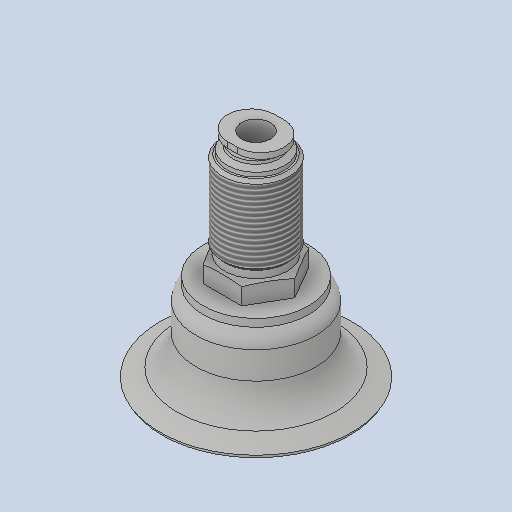
# Autodesk Inventor part: MVFKN40-1-1
Saved by Autodesk Inventor 2024.1 (Build 281209000, 209)
## iProperties
Category: PARTsolutions
Company: MISUMI
Created: 2023-12-16
Part Number: MVFKN40-1-1
Material: Generic
Catalog Web Link: www.cadenas.de
Description: MVPKN, MVPKE, MVPKF, MVFKN, MVFKF,MVSKS_1-Suction Cups - StandardType, Deep Type, Sponge Type - Fixed Type Up: One  - Touch Type (K Shape)_1
Vendor: MISUMI
Document SubType Name: Modeling
Designer: psAdmin
Manufacturer: MISUMI
Mass: 14.6095 g
Surface Area: 52.8765 cm^2
Volume: 14.6095 cm^3
Density: 1 g/cm^3
Appearance: PSOLRGB-175-175-175
PSOL_IDENT_0: {$CADENAS_DATA/23d-libs/misumi/metric/35_tubes_nozzles/mvpkn/mvpkn.prj},200 {VTYP=3D},{NB=MVFKN40-1-
PSOL_IDENT_1: 1},{LINA=MVFKN40-1},{NN=MVPKN, MVPKE, MVPKF, MVFKN, MVFKF,MVSKS_1},{DATE=04.06.2021 06:55:05},{GEOMD
PSOL_IDENT_2: ATE=14.07.2014 08:56:00},{VERSION=},{LINEID=120},{WBVAR=MATP},{WBNUMERIC=}  {NB=MVFKN40-1-1},{LINA=M
PSOL_IDENT_3: VFKN40-1},{KT=DUMMY},{PN=MVFKN40-1},{MATM=Brass},{TYPE=MVFKN},{ST=Electroless Nickel Plating},{AC=Su
PSOL_IDENT_4: ction Cup},{SHAPE=Deep},{MATP=N},{MATPALG='N', 'Nitrile Rubber','F','Fluoro Rubber'},{NL1=40 - 17.5}
PSOL_IDENT_5: ,{NO=40},{NO1=40},{D=6},{DD=40},{L1=17.5},{B=45.2},{L2=23.1},{L3=18.0},{H1=17},{T=4},{M=M14x1.0},{M1=
PSOL_IDENT_6: 14},{M2=1.00},{L4=11.7},{MASS=47.0},{TIFF=2},{MVPNT=1},{MVPFT=1},{K1=0},{K2=0},{K3=0.0},{MVPKN=1},{P
PSOL_IDENT_7: LANE=17.500},{R1=4.9},{H2=7.0},{H3=9.5},{H4=12.0},{L5=0.0},{L6=1.5},{H5=22.0},{H6=14},{VD1=40},{VD2=
PSOL_IDENT_8: 25.0},{VD3=0.0},{VH1=17.5},{VH2=4.5},{VX1=0.00},{VX2=0.0},{VY1=0.77},{VY2=0.0},{VY3=0.00},{VR1=7.00}
NB: MVFKN40-1-1
NN: MVPKN, MVPKE, MVPKF, MVFKN, MVFKF,MVSKS_1
NT: Suction Cups - StandardType, Deep Type, Sponge Type - Fixed Type Up: One  - Touch Type (K Shape)_1
NBSYN: $PN.-1
LINA: MVFKN40-1
CATALOG: Misumi
PN: MVFKN40-1
MATM: Brass
ST: Electroless Nickel Plating
AC: Suction Cup
SHAPE: Deep
MATP: Nitrile Rubber
NL1: 40 - 17.5
NO: 40
D: 6
DD: 40
L1: 17.5
B: 45.2
L2: 23.1
L3: 18
H1: 17
T: 4
M: M14x1.0
M2: 1
MASS: 47
K1: 0
K2: 0
K3: 0
PLANE: 17.5
R1: 4.9
H2: 7
H3: 9.5
H4: 12
L5: 0
L6: 1.5
H5: 22
H6: 14
VD1: 40
VD2: 25
VD3: 0
VH1: 17.5
VH2: 4.5
VX1: 0
VX2: 0
VY1: 0.77
VY2: 0
VY3: 0
VR1: 7
SUPPLIER: MISUMI
ARTICLENO: MVFKN40-1-1
BOMINFO: MVFKN40-1
CREATOR: CADENAS GmbH
Title: MVFKN40-1
Author: Cadenas PARTsolutions
Comments: Suction Cups - StandardType, Deep Type, Sponge Type - Fixed Type Up: One  - Touch Type (K Shape)_1
Autodesk Inventor part; units mm, degrees
sketch "Sketch_1" plane through (0, 45.2, 0) normal (0, 1, 0) x (1, 0, 0)
  arc A0 (-1, 4.9) -> (-1, -4.9) centre (-1, 0) ccw
  line L0 (-1, -4.9) -> (1, -4.9)
  arc A1 (1, -4.9) -> (1, 4.9) centre (1, 0) ccw
  line L1 (1, 4.9) -> (-1, 4.9)
  constraints: 4 end point, 4 point on circle, 2 centre point
extrude "Extrusion1" add sketch "Sketch_1" against normal blind 1.2
sketch "Sketch_2" plane through (0, 0, 0) normal (0, 0, 1) x (1, 0, 0)
  line L0 (0, 41.1) -> (0, 44)
  line L1 (0, 44) -> (3.5, 44)
  line L2 (3.5, 44) -> (3.5, 43.1)
  line L3 (3.5, 43.1) -> (4.75, 43.1)
  line L4 (4.75, 43.1) -> (4.884, 42.6)
  line L5 (4.884, 42.6) -> (6, 41.9557)
  line L6 (6, 41.9557) -> (6, 41.1)
  line L7 (6, 41.1) -> (0, 41.1)
  line L8 (0, 41.1) -> (0, 44)
  constraints: 18 end point
revolve "Revolution1" add sketch "Sketch_2" angle 360 about axis through (0, 41.1, 0) along (0, -1, 0)
sketch "Sketch_5" plane through (0, 0, 0) normal (0, 0, 1) x (1, 0, 0)
  line L0 (0, 24.6) -> (0, 41.1)
  line L1 (0, 41.1) -> (6.3865, 41.1)
  line L2 (6.3865, 41.1) -> (7, 40.4865)
  line L3 (7, 40.4865) -> (7, 25.2135)
  line L4 (7, 25.2135) -> (6.3865, 24.6)
  line L5 (6.3865, 24.6) -> (0, 24.6)
  line L6 (0, 24.6) -> (0, 41.1)
  constraints: 14 end point
revolve "Revolution2" add sketch "Sketch_5" angle 360 about axis through (0, 24.6, 0) along (0, -1, 0)
thread "Thread1" size "M14x1" class "6g" standard "ISO Metric profile" full length
sketch "Sketch_6" plane through (0, 0, 0) normal (0, 0, 1) x (1, 0, 0)
  line L0 (0, 23.1) -> (0, 24.6)
  line L1 (0, 24.6) -> (6.5, 24.6)
  line L2 (6.5, 24.6) -> (6.5, 23.1)
  line L3 (6.5, 23.1) -> (0, 23.1)
  line L4 (0, 23.1) -> (0, 24.6)
  constraints: 10 end point
revolve "Revolution3" add sketch "Sketch_6" angle 360 about axis through (0, 23.1, 0) along (0, -1, 0)
sketch "Sketch_8" plane through (0, 0, 0) normal (0, 0, 1) x (1, 0, 0)
  line L0 (0, 17.5) -> (0, 23.1)
  line L1 (0, 23.1) -> (6, 23.1)
  line L2 (6, 23.1) -> (8.4, 22.4569)
  line L3 (8.4, 22.4569) -> (8.4, 18.1431)
  line L4 (8.4, 18.1431) -> (6, 17.5)
  line L5 (6, 17.5) -> (0, 17.5)
  line L6 (0, 17.5) -> (0, 23.1)
  constraints: 14 end point
revolve "Revolution4" add sketch "Sketch_8" angle 360 about axis through (0, 17.5, 0) along (0, -1, 0)
sketch "Sketch_9" plane through (0, 23.1, 0) normal (0, 1, 0) x (1, 0, 0)
  line L0 (-12, -12) -> (12, -12)
  line L1 (12, -12) -> (12, 12)
  line L2 (12, 12) -> (-12, 12)
  line L3 (-12, 12) -> (-12, -12)
  line L4 (-8.0829, 0) -> (-4.0415, -7)
  line L5 (-4.0415, -7) -> (4.0415, -7)
  line L6 (4.0415, -7) -> (8.0829, 0)
  line L7 (8.0829, 0) -> (4.0415, 7)
  line L8 (4.0415, 7) -> (-4.0415, 7)
  line L9 (-4.0415, 7) -> (-8.0829, 0)
  constraints: 20 end point
extrude "Extrusion2" cut sketch "Sketch_9" against normal blind 5.6
sketch "Sketch_10" plane through (0, 0, 0) normal (0, 0, 1) x (1, 0, 0)
  line L0 (0, 17.5) -> (0, 19.1)
  line L1 (0, 19.1) -> (11, 19.1)
  line L2 (11, 19.1) -> (11, 17.5)
  line L3 (11, 17.5) -> (0, 17.5)
  line L4 (0, 17.5) -> (0, 19.1)
  constraints: 10 end point
revolve "Revolution5" add sketch "Sketch_10" angle 360 about axis through (0, 17.5, 0) along (0, -1, 0)
sketch "Sketch_12" plane through (0, 0, 0) normal (0, 0, 1) x (1, 0, 0)
  line L0 (0, 33.5) -> (0, 45.2)
  line L1 (0, 45.2) -> (3, 45.2)
  line L2 (3, 45.2) -> (3, 33.5)
  line L3 (3, 33.5) -> (0, 33.5)
  line L4 (0, 33.5) -> (0, 45.2)
  constraints: 10 end point
revolve "Revolution6" cut sketch "Sketch_12" angle 360 about axis through (0, 33.5, 0) along (0, -1, 0)
sketch "Sketch_22" plane through (0, 0, 0) normal (0, 0, 1) x (1, 0, 0)
  line L0 (0, 17.5) -> (0, 0)
  line L1 (0, 0) -> (-19.5554, 0)
  line L2 (-19.5554, 0) -> (-20, 0.77)
  line L3 (-20, 0.77) -> (-16.3829, 2.5689)
  arc A0 (-16.3829, 2.5689) -> (-12.5, 8.8366) centre (-19.5, 8.8366) ccw
  line L4 (-12.5, 8.8366) -> (-12.5, 14.5)
  arc A1 (-9.5, 17.5) -> (-12.5, 14.5) centre (-9.5, 14.5) ccw
  line L5 (-9.5, 17.5) -> (0, 17.5)
  line L6 (0, 17.5) -> (0, 0)
  constraints: 14 end point, 4 point on circle, 2 centre point
revolve "Revolution7" add sketch "Sketch_22" angle 360 about axis through (0, 17.5, 0) along (0, 1, 0)
ref_plane "BODY_TO_PARTS_XY" through (0, 17.5, 0) normal (0, 1, 0) x (1, 0, 0)
ref_plane "BODY_TO_PARTS_YZ" through (0, 17.5, 0) normal (1, 0, 0) x (0, 0, -1)
ref_plane "BODY_TO_PARTS_ZX" through (0, 17.5, 0) normal (0, 0, -1) x (0, 1, 0)
ref_plane "body_to_nut1_XY" through (0, 30.3, 0) normal (0, 1, 0) x (1, 0, 0)
ref_plane "body_to_nut1_YZ" through (0, 30.3, 0) normal (1, 0, 0) x (0, 0, -1)
ref_plane "body_to_nut1_ZX" through (0, 30.3, 0) normal (0, 0, -1) x (0, 1, 0)
ref_plane "body_to_nut2_XY" through (0, 24.7, 0) normal (0, 1, 0) x (1, 0, 0)
ref_plane "body_to_nut2_YZ" through (0, 24.7, 0) normal (1, 0, 0) x (0, 0, -1)
ref_plane "body_to_nut2_ZX" through (0, 24.7, 0) normal (0, 0, -1) x (0, 1, 0)
ref_plane "body_to_nut3_XY" through (0, 34.6, 0) normal (0, 1, 0) x (1, 0, 0)
ref_plane "body_to_nut3_YZ" through (0, 34.6, 0) normal (1, 0, 0) x (0, 0, -1)
ref_plane "body_to_nut3_ZX" through (0, 34.6, 0) normal (0, 0, -1) x (0, 1, 0)
ref_plane "body_to_nut4_XY" through (0, 27.6, 0) normal (0, 1, 0) x (1, 0, 0)
ref_plane "body_to_nut4_YZ" through (0, 27.6, 0) normal (1, 0, 0) x (0, 0, -1)
ref_plane "body_to_nut4_ZX" through (0, 27.6, 0) normal (0, 0, -1) x (0, 1, 0)
ref_plane "作業平面17" through (0, 0, 10) normal (0, 0, 1) x (1, 0, 0)
sketch "スケッチ11" plane through (0, 0, 10) normal (0, 0, 1) x (1, 0, 0)
  arc A0 (-16.3829, 2.5689) -> (-12.5, 8.8366) centre (-19.5, 8.8366) ccw projected
  line L0 (0, 0) -> (-19.5554, 0) projected
  line L1 (-19.5554, 0) -> (-20, 0.77) projected
  line L2 (-5.9, 44) -> (-1, 44) projected
  line L3 (-1, 45.2) -> (-5.9, 45.2) projected
  line L4 (-1, 45.2) -> (-1, 44) projected
  line L5 (-4.884, 42.6) -> (4.884, 42.6) projected
  line L6 (-4.884, 42.6) -> (4.884, 42.6) projected
  line L7 (-4.75, 43.1) -> (4.75, 43.1) projected
  line L8 (-3.5, 43.1) -> (3.5, 43.1) projected
  line L9 (-4.75, 43.1) -> (4.75, 43.1) projected
  line L10 (-1, 44) -> (1, 44) projected
  line L11 (1, 44) -> (-1, 44) projected
  line L12 (3.5, 44) -> (-3.5, 44) projected
  line L13 (-3.5, 43.1) -> (3.5, 43.1) projected
  line L14 (3.5, 44) -> (-3.5, 44) projected
  line L15 (1, 44) -> (5.9, 44) projected
  line L16 (3.5, 44) -> (-3.5, 44) projected
  line L17 (-1, 44) -> (-1, 44) projected
  line L18 (-1, 44) -> (1, 44) projected
  line L19 (1, 44) -> (1, 44) projected
  line L20 (1, 44) -> (-1, 44) projected
  line L21 (-3, 45.2) -> (3, 45.2) projected
  line L22 (-1, 45.2) -> (-1, 45.2) projected
  line L23 (-1, 45.2) -> (1, 45.2) projected
  line L24 (1, 45.2) -> (1, 45.2) projected
  line L25 (1, 45.2) -> (-1, 45.2) projected
  line L26 (5.9, 45.2) -> (1, 45.2) projected
  line L27 (1, 45.2) -> (1, 45.2) projected
  line L28 (1, 45.2) -> (1, 44) projected
  line L29 (1, 44) -> (1, 44) projected
  line L30 (1, 45.2) -> (1, 44) projected
  line L31 (1, 45.2) -> (1, 44) projected
  line L32 (-1, 45.2) -> (1, 45.2) projected
  line L33 (-1, 45.2) -> (1, 45.2) projected
  line L34 (-1, 45.2) -> (-1, 44) projected
  line L35 (1, 44) -> (-1, 44) projected
  line L36 (1, 45.2) -> (1, 44) projected
  line L37 (1, 45.2) -> (-1, 45.2) projected
  line L38 (1, 45.2) -> (1, 44) projected
  line L39 (1, 45.2) -> (-1, 45.2) projected
  line L40 (1, 45.2) -> (1, 44) projected
  line L41 (-1, 44) -> (1, 44) projected
  line L42 (-1, 45.2) -> (-1, 44) projected
  line L43 (-3, 45.2) -> (3, 45.2) projected
  line L44 (-4.75, 43.1) -> (4.75, 43.1) projected
  line L45 (-3.5, 43.1) -> (3.5, 43.1) projected
  line L46 (-3, 33.5) -> (3, 33.5) projected
  line L47 (-3, 45.2) -> (3, 45.2) projected
  line L48 (-6, 41.9557) -> (6, 41.9557) projected
  line L49 (-4.884, 42.6) -> (4.884, 42.6) projected
  line L50 (-6, 41.9557) -> (6, 41.9557) projected
  line L51 (-6, 41.1) -> (6, 41.1) projected
  line L52 (-6, 41.9557) -> (6, 41.9557) projected
  line L53 (-6, 41.1) -> (6, 41.1) projected
  line L54 (-3, 33.5) -> (3, 33.5) projected
  line L55 (-3, 33.5) -> (3, 33.5) projected
  line L56 (-6.3865, 41.1) -> (6.3865, 41.1) projected
  line L57 (-6.3865, 41.1) -> (6.3865, 41.1) projected
  line L58 (-6, 41.1) -> (6, 41.1) projected
  line L59 (-7, 40.4865) -> (7, 40.4865) projected
  line L60 (-7, 25.2135) -> (7, 25.2135) projected
  line L61 (-7, 40.4865) -> (7, 40.4865) projected
  line L62 (-7, 40.4865) -> (7, 40.4865) projected
  line L63 (-6.3865, 41.1) -> (6.3865, 41.1) projected
  line L64 (-7, 25.2135) -> (7, 25.2135) projected
  line L65 (-6.5, 23.1) -> (6.5, 23.1) projected
  line L66 (-6.3865, 24.6) -> (6.3865, 24.6) projected
  line L67 (-6.5, 24.6) -> (6.5, 24.6) projected
  line L68 (6, 23.1) -> (-6, 23.1) projected
  line L69 (-8.0829, 22.5419) -> (-8.0829, 19.1) projected
  line L70 (-4.0415, 22.5419) -> (-4.0415, 19.1) projected
  line L71 (4.0415, 22.5419) -> (4.0415, 19.1) projected
  line L72 (8.0829, 22.5419) -> (8.0829, 19.1) projected
  line L73 (-4.0415, 22.5419) -> (-4.0415, 19.1) projected
  line L74 (4.0415, 22.5419) -> (4.0415, 19.1) projected
  line L75 (4.0415, 19.1) -> (-4.0415, 19.1) projected
  line L76 (4.0415, 19.1) -> (-4.0415, 19.1) projected
  line L77 (-4.0415, 22.5419) -> (-4.0415, 19.1) projected
  line L78 (4.0415, 22.5419) -> (4.0415, 19.1) projected
  line L79 (-6.5, 24.6) -> (6.5, 24.6) projected
  line L80 (-6.3865, 24.6) -> (6.3865, 24.6) projected
  line L81 (-6.3865, 24.6) -> (6.3865, 24.6) projected
  line L82 (-7, 25.2135) -> (7, 25.2135) projected
  line L83 (-6.5, 23.1) -> (6.5, 23.1) projected
  line L84 (-6.5, 24.6) -> (6.5, 24.6) projected
  line L85 (-4.0415, 19.1) -> (-8.0829, 19.1) projected
  line L86 (8.0829, 19.1) -> (4.0415, 19.1) projected
  line L87 (8.0829, 19.1) -> (4.0415, 19.1) projected
  line L88 (4.0415, 22.5419) -> (4.0415, 19.1) projected
  line L89 (8.0829, 22.5419) -> (8.0829, 19.1) projected
  line L90 (-4.0415, 19.1) -> (-8.0829, 19.1) projected
  line L91 (-8.0829, 22.5419) -> (-8.0829, 19.1) projected
  line L92 (-4.0415, 22.5419) -> (-4.0415, 19.1) projected
  line L93 (-8.0829, 19.1) -> (-4.0415, 19.1) projected
  line L94 (-8.0829, 19.1) -> (-4.0415, 19.1) projected
  line L95 (-4.0415, 22.5419) -> (-4.0415, 19.1) projected
  line L96 (-8.0829, 22.5419) -> (-8.0829, 19.1) projected
  line L97 (6, 23.1) -> (-6, 23.1) projected
  line L98 (-4.0415, 19.1) -> (4.0415, 19.1) projected
  line L99 (-4.0415, 19.1) -> (4.0415, 19.1) projected
  line L100 (4.0415, 22.5419) -> (4.0415, 19.1) projected
  line L101 (-4.0415, 22.5419) -> (-4.0415, 19.1) projected
  line L102 (6, 23.1) -> (-6, 23.1) projected
  line L103 (-6.5, 23.1) -> (6.5, 23.1) projected
  line L104 (4.0415, 19.1) -> (8.0829, 19.1) projected
  line L105 (4.0415, 19.1) -> (8.0829, 19.1) projected
  line L106 (8.0829, 22.5419) -> (8.0829, 19.1) projected
  line L107 (4.0415, 22.5419) -> (4.0415, 19.1) projected
  line L108 (-1, 45.2) -> (-1, 44) projected
  line L109 (-1, 45.2) -> (-1, 45.2) projected
  line L110 (-1, 45.2) -> (-1, 44) projected
  line L111 (-1, 44) -> (-1, 44) projected
  line L112 (-1, 45.2) -> (-1, 44) projected
  line L113 (-11, 19.1) -> (11, 19.1) projected
  line L114 (-11, 17.5) -> (11, 17.5) projected
  line L115 (-9.5, 17.5) -> (9.5, 17.5) projected
  line L116 (12.5, 14.5) -> (-12.5, 14.5) projected
  line L117 (12.5, 8.8366) -> (-12.5, 8.8366) projected
  line L118 (-11, 19.1) -> (11, 19.1) projected
  line L119 (4.0415, 19.1) -> (-4.0415, 19.1) projected
  line L120 (8.0829, 19.1) -> (4.0415, 19.1) projected
  line L121 (4.0415, 19.1) -> (8.0829, 19.1) projected
  line L122 (-4.0415, 19.1) -> (4.0415, 19.1) projected
  line L123 (-8.0829, 19.1) -> (-4.0415, 19.1) projected
  line L124 (-4.0415, 19.1) -> (-8.0829, 19.1) projected
  line L125 (-11, 17.5) -> (11, 17.5) projected
  line L126 (-11, 19.1) -> (11, 19.1) projected
  line L127 (-9.5, 17.5) -> (9.5, 17.5) projected
  line L128 (12.5, 14.5) -> (-12.5, 14.5) projected
  line L129 (12.5, 14.5) -> (-12.5, 14.5) projected
  line L130 (12.5, 8.8366) -> (-12.5, 8.8366) projected
  line L131 (-11, 17.5) -> (11, 17.5) projected
  line L132 (-9.5, 17.5) -> (9.5, 17.5) projected
  line L133 (0, 17.5) -> (0, 19.1) projected
  line L134 (0, 19.1) -> (11, 19.1) projected
  line L135 (11, 19.1) -> (11, 17.5) projected
  line L136 (11, 17.5) -> (0, 17.5) projected
  line L137 (0, 17.5) -> (0, 19.1) projected
  line L138 (0, 33.5) -> (0, 45.2) projected
  line L139 (0, 45.2) -> (3, 45.2) projected
  line L140 (3, 45.2) -> (3, 33.5) projected
  line L141 (3, 33.5) -> (0, 33.5) projected
  line L142 (0, 33.5) -> (0, 45.2) projected
  line L143 (0, 17.5) -> (0, 0) projected
  line L144 (-20, 0.77) -> (-16.3829, 2.5689) projected
  line L145 (-12.5, 8.8366) -> (-12.5, 14.5) projected
  arc A1 (-9.5, 17.5) -> (-12.5, 14.5) centre (-9.5, 14.5) ccw projected
  line L146 (-9.5, 17.5) -> (0, 17.5) projected
  line L147 (0, 17.5) -> (0, 0) projected
  line L148 (0, 17.5) -> (0, 23.1) projected
  line L149 (0, 23.1) -> (6, 23.1) projected
  line L150 (6, 23.1) -> (8.4, 22.4569) projected
  line L151 (8.4, 22.4569) -> (8.4, 18.1431) projected
  line L152 (8.4, 18.1431) -> (6, 17.5) projected
  line L153 (6, 17.5) -> (0, 17.5) projected
  line L154 (0, 17.5) -> (0, 23.1) projected
  line L155 (0, 23.1) -> (0, 24.6) projected
  line L156 (0, 24.6) -> (6.5, 24.6) projected
  line L157 (6.5, 24.6) -> (6.5, 23.1) projected
  line L158 (6.5, 23.1) -> (0, 23.1) projected
  line L159 (0, 23.1) -> (0, 24.6) projected
  line L160 (0, 24.6) -> (0, 41.1) projected
  line L161 (0, 41.1) -> (6.3865, 41.1) projected
  line L162 (6.3865, 41.1) -> (7, 40.4865) projected
  line L163 (7, 40.4865) -> (7, 25.2135) projected
  line L164 (7, 25.2135) -> (6.3865, 24.6) projected
  line L165 (6.3865, 24.6) -> (0, 24.6) projected
  line L166 (0, 24.6) -> (0, 41.1) projected
  line L167 (0, 41.1) -> (0, 44) projected
  line L168 (0, 44) -> (3.5, 44) projected
  line L169 (3.5, 44) -> (3.5, 43.1) projected
  line L170 (3.5, 43.1) -> (4.75, 43.1) projected
  line L171 (4.75, 43.1) -> (4.884, 42.6) projected
  line L172 (4.884, 42.6) -> (6, 41.9557) projected
  line L173 (6, 41.9557) -> (6, 41.1) projected
  line L174 (6, 41.1) -> (0, 41.1) projected
  line L175 (0, 41.1) -> (0, 44) projected
  constraints: 18 horizontal alignment, 23 other
body "Solid1"
